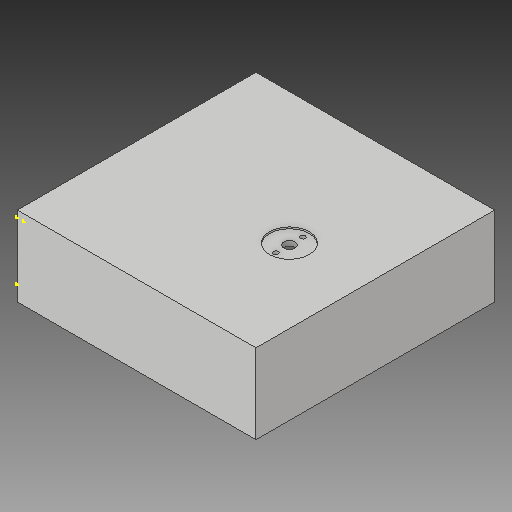
# Autodesk Inventor part: base sup
Saved by Autodesk Inventor 2018.2 (Build 222227000, 227)
## iProperties
Created: 2016-05-12
Part Number: base sup
Material: Genérico
Document SubType Name: Modeling
Designer: Usuario
Density: 1 g/cm^3
Appearance: Valor por defecto
Author: Usuario
Autodesk Inventor part; units mm, degrees
ref_plane "YZ Plane" through (0, 0, 0) normal (1, 0, 0) x (0, 1, 0)
ref_plane "XZ Plane" through (0, 0, 0) normal (0, 1, 0) x (-1, 0, 0)
ref_plane "XY Plane" through (0, 0, 0) normal (0, 0, 1) x (1, 0, 0)
sketch "Boceto1" plane through (0, 0, 0) normal (0, 1, 0) x (-1, 0, 0)
  line L0 (0, 0) -> (0, -150)
  line L1 (0, -150) -> (-150, -150)
  line L2 (-150, -150) -> (-150, 0)
  line L3 (-150, 0) -> (0, 0)
  constraints: 8 end point, 2 perpendicular, 1 vertical
extrude "Extrusión1" add sketch "Boceto1" along normal blind 4
sketch "Boceto2" plane through (0, 4, 0) normal (0, 1, 0) x (1, 0, 0)
  line L0 (0, 0) -> (150, 0) projected
  circle A0 centre (103.5, 67.5) radius 12.5
  constraints: 1 centre point
extrude "Extrusión2" cut sketch "Boceto2" against normal blind 1
sketch "Boceto3" plane through (0, 4, 0) normal (0, 1, 0) x (1, 0, 0)
  circle A0 centre (103.5, 67.5) radius 12.5 projected
  circle A1 centre (103.5, 76) radius 1.5
  circle A2 centre (103.5, 59) radius 1.5
  circle A3 centre (103.5, 67.5) radius 3.5
  point P0 (0, 0)
  constraints: 3 centre point, 1 coincident
extrude "Extrusión3" cut sketch "Boceto3" against normal blind 4 contours A1 | A2 | A3
sketch "Boceto4" plane through (0, 0, 0) normal (0, -1, 0) x (1, 0, 0)
  point P0 (0, 0)
sketch "Boceto5" plane through (0, 0, 0) normal (0, -1, 0) x (1, 0, 0)
  line L0 (0, 0) -> (0, -4)
  line L1 (150, -4) -> (150, 0)
  line L2 (150, 0) -> (0, 0)
  line L3 (4, -4) -> (146, -4)
  line L4 (0, 0) -> (4, 0)
  line L5 (0, 0) -> (150, 0) projected
  line L6 (4, -4) -> (4, -146)
  line L7 (0, -150) -> (0, 0) projected
  line L8 (0, -4) -> (0, -150)
  line L9 (0, -150) -> (150, -150)
  line L10 (150, -150) -> (150, -4)
  line L11 (0, -150) -> (0, -146)
  line L12 (4, -146) -> (146, -146)
  line L13 (150, -150) -> (146, -150)
  line L14 (150, -150) -> (0, -150) projected
  line L15 (146, -146) -> (146, -4)
  constraints: 26 end point, 5 perpendicular, 3 point on line, 2 vertical, 1 horizontal
extrude "Extrusión4" add sketch "Boceto5" along normal blind 46
sketch "Boceto6" plane through (0, -46, 0) normal (0, -1, 0) x (1, 0, 0)
  line L0 (4, -4) -> (4, -146)
  line L1 (4, -146) -> (146, -146) projected
  line L2 (4, -146) -> (146, -146)
  line L3 (146, -146) -> (146, -4)
  line L4 (146, -4) -> (4, -4)
  line L5 (1.7, -4) -> (1.7, -148.3)
  line L6 (1.7, -148.3) -> (148.3, -148.3)
  line L7 (150, -150) -> (0, -150) projected
  line L8 (146, -1.7) -> (1.7, -1.7)
  line L9 (1.7, -4) -> (1.7, -1.7)
  line L10 (146, -1.7) -> (148.3, -1.7)
  line L11 (148.3, -1.7) -> (148.3, -148.3)
  point P0 (0, 0)
  constraints: 20 end point, 5 perpendicular, 1 horizontal, 1 parallel, 1 vertical
extrude "Extrusión5" cut sketch "Boceto6" against normal blind 10
sketch "Boceto7" plane through (0, -36, 0) normal (0, -1, 0) x (1, 0, 0)
  point P0 (0, 0)
sketch "Boceto8" plane through (4, 0, -4) normal (1, 0, 0) x (0, 0, -1)
  point P0 (-4, 0)
sketch "Boceto9" plane through (0, 4, -150) normal (-1, 0, 0) x (0, 0, 1)
  line L0 (150, -50) -> (146, -50)
  line L1 (150, -50) -> (150, 0)
  line L2 (150, 0) -> (0, 0)
  line L3 (150, -50) -> (0, -50) projected
  line L4 (0, 0) -> (0, -50)
  line L5 (0, -50) -> (4, -50)
  line L6 (0, 0) -> (0, -4)
  line L7 (4, 0) -> (146, 0)
  line L8 (150, 0) -> (146, 0)
  line L9 (0, 0) -> (150, 0) projected
  line L10 (146, 0) -> (146, -50)
  line L11 (0, 0) -> (4, 0)
  line L12 (4, 0) -> (4, -50)
  line L13 (4, -50) -> (146, -50)
  point P0 (150, -4)
  constraints: 24 end point, 4 perpendicular, 4 point on line, 2 horizontal, 1 collinear, 1 vertical
extrude "Extrusión6" cut sketch "Boceto9" against normal blind 4 contours L3 L12 L2 L10
sketch "Boceto10" plane through (0, 4, 0) normal (0, 0, 1) x (1, 0, 0)
  point P0 (0, -4)
sketch "Boceto11" plane through (4, 4, -150) normal (-1, 0, 0) x (0, 0, 1)
  line L0 (146, -4) -> (4, -4) projected
  line L1 (146, -4) -> (146, -40) projected
  line L2 (4, -4) -> (146, -4)
  line L3 (146, 0) -> (150, 0) projected
  line L4 (146, -4) -> (146, 0)
  line L5 (146, 0) -> (4, 0)
  line L6 (4, 0) -> (4, -4)
  point P0 (150, -4)
  constraints: 8 end point, 3 perpendicular, 1 horizontal
extrude "Extrusión7" add sketch "Boceto11" along normal blind 4
sketch "Boceto12" plane through (0, 4, 0) normal (0, 0, 1) x (1, 0, 0)
  point P0 (0, -4)
